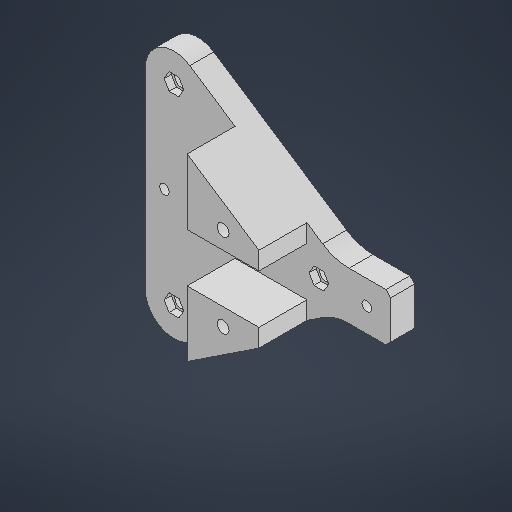
# Autodesk Inventor part: y axis something back
Saved by Autodesk Inventor 2025.1 (Build 291241000, 241)
## iProperties
Created: 2025-02-02
Part Number: y axis something back
Material: Generic
Document SubType Name: Modeling
Designer: jerem
Density: 1 g/cm^3
Appearance: Default
Author: jerem
## iProperties of the stored document y axis something back_3DPrint.ipt
Created: 2025-02-19
Part Number: y axis something back_3DPrint
Material: Generic
Document SubType Name: Modeling
Designer: jerem
Density: 1 g/cm^3
Appearance: Default
Author: jerem
Autodesk Inventor part; units mm, degrees
ref_plane "YZ Plane" through (0, 0, 0) normal (1, 0, 0) x (0, 1, 0)
ref_plane "XZ Plane" through (0, 0, 0) normal (0, 1, 0) x (-1, 0, 0)
ref_plane "XY Plane" through (0, 0, 0) normal (0, 0, 1) x (1, 0, 0)
sketch "Sketch1" plane through (0, 0, 0) normal (0, 0, 1) x (1, 0, 0)
  line L0 (0, 0) -> (30.25, 0) construction
  line L1 (0, 0) -> (-30.25, 0) construction
  line L2 (-30.25, 0) -> (-30.25, 40) construction
  line L3 (-30.25, 0) -> (-30.25, -40) construction
  circle A0 centre (-30.25, 40) radius 2.7
  circle A1 centre (-30.25, -40) radius 2.7
  circle A2 centre (30.25, 0) radius 2.7
  circle A3 centre (-30.25, 40) radius 12
  circle A4 centre (-30.25, -40) radius 12
  circle A5 centre (30.25, 0) radius 12
  line L4 (36.868172, -10.009985) -> (-23.631828, -50.009985)
  line L5 (-42.25, 40) -> (-42.25, -40)
  circle A6 centre (-34.25, 0) radius 2
  line L6 (-30.25, 0) -> (-34.25, 0) construction
  line L7 (-23.631828, 50.009985) -> (36.868172, 10.009985)
  line L8 (30.25, 0) -> (50.25, 0) construction
  circle A7 centre (50.25, 0) radius 10
  circle A8 centre (50.25, 0) radius 2
  line L9 (50.25746, 9.999997) -> (36.868172, 10.009985)
  line L10 (50.25746, -9.999997) -> (36.868172, -10.009985)
  circle A9 centre (10.25, 0) radius 2
  line L11 (50.25746, -9.999997) -> (60.257457, -9.992538)
  line L12 (60.257457, -9.992538) -> (60.242549, 9.992549)
  line L13 (60.242549, 9.992549) -> (50.25746, 9.999997)
  point P0 (-42.25, 0)
  point P1 (41.35, -4.559605)
  point P2 (41.35, 4.559605)
  point P3 (60.249997, 0.00746)
  dimension "d0" = 60.5
  dimension "d1" = 5.4
  dimension "d2" = 80
  dimension "d3" = 24
  dimension "d55" = 4
  dimension "d56" = 8
  dimension "d57" = 20
  dimension "d58" = 20
  dimension "d69" = 20
  constraints: 28 end point, 10 centre point, 10 tangent, 8 coincident, 8 point on circle, 6 equal radius, 4 horizontal, 2 collinear, 2 perpendicular, 2 vertical, 1 midpoint, 1 point on line
  measures "d0" distance of L0.end L1.end
  measures "d1" diameter of A0
  measures "d2" distance of L3.end L2.end
  measures "d3" diameter of A3
  measures "d55" diameter of A6
  measures "d56" distance of point (-42.25, 0) L6.end
  measures "d57" distance of L8.start L8.end
  measures "d58" diameter of A7
  measures "d69" distance of A9.centre L0.end
sketch "Sketch1 outline for Extrusion1" plane through (0, 0, 0) normal (0, 0, 1) x (1, 0, 0)
  arc A0 (-23.631828, 50.009985) -> (-42.25, 40) centre (-30.25, 40) ccw
  line L0 (-42.25, 40) -> (-42.25, -40)
  arc A1 (-42.25, -40) -> (-23.631828, -50.009985) centre (-30.25, -40) ccw
  line L1 (-23.631828, -50.009985) -> (36.868172, -10.009985)
  line L2 (36.868172, -10.009985) -> (60.257457, -9.992538)
  line L3 (60.257457, -9.992538) -> (60.242549, 9.992549)
  line L4 (60.242549, 9.992549) -> (36.868172, 10.009985)
  line L5 (36.868172, 10.009985) -> (-23.631828, 50.009985)
  circle A2 centre (-30.25, 40) radius 2.7
  circle A3 centre (10.25, 0) radius 2
  circle A4 centre (-34.25, 0) radius 2
  circle A5 centre (30.25, 0) radius 2.7
  circle A6 centre (-30.25, -40) radius 2.7
  circle A7 centre (50.25, 0) radius 2
extrude "Extrusion1" add sketch "Sketch1 outline for Extrusion1" against normal blind 10
fillet "Fillet1" radius 20 2 edges at (36.8682, 10.01, -5) (36.8682, -10.01, -5)
chamfer "Chamfer6" distance 2 angle 45 2 edges at (60.2425, 9.9925, -5) (60.2575, -9.9925, -5)
sketch "Sketch8" plane through (0, 0, 0) normal (0, 0, 1) x (1, 0, 0)
  line L0 (58.257457, -9.99403) -> (60.255965, -7.992538)
  line L1 (58.257457, -9.99403) -> (42.873828, -10.005505)
  arc A0 (42.873828, -10.005505) -> (31.85846, -13.322191) centre (42.888747, -30.0055) ccw
  line L2 (31.85846, -13.322191) -> (-23.631828, -50.009985)
  arc A1 (-42.25, -40) -> (-23.631828, -50.009985) centre (-30.25, -40) ccw
  line L3 (-42.25, -40) -> (-42.25, 40)
  arc A2 (-23.631828, 50.009985) -> (-42.25, 40) centre (-30.25, 40) ccw
  line L4 (-23.631828, 50.009985) -> (31.85846, 13.322191)
  arc A3 (31.85846, 13.322191) -> (42.873828, 10.005505) centre (42.888747, 30.0055) ccw
  line L5 (42.873828, 10.005505) -> (58.242549, 9.994041)
  line L6 (60.244041, 7.992549) -> (58.242549, 9.994041)
  line L7 (60.244041, 7.992549) -> (60.255965, -7.992538)
  circle A4 centre (30.25, 0) radius 2.7
  circle A5 centre (50.25, 0) radius 2
  circle A6 centre (-30.25, -40) radius 2.7
  circle A7 centre (-34.25, 0) radius 2
  circle A8 centre (10.25, 0) radius 2
  circle A9 centre (-30.25, 40) radius 2.7
  line L8 (-28.200407, -43.55) -> (-32.299593, -43.55)
  line L9 (-32.299593, -43.55) -> (-34.349187, -40)
  line L10 (-34.349187, -40) -> (-32.299593, -36.45)
  line L11 (-32.299593, -36.45) -> (-28.200407, -36.45)
  line L12 (-28.200407, -36.45) -> (-26.150813, -40)
  line L13 (-26.150813, -40) -> (-28.200407, -43.55)
  line L14 (-28.200407, 36.45) -> (-32.299593, 36.45)
  line L15 (-32.299593, 36.45) -> (-34.349187, 40)
  line L16 (-34.349187, 40) -> (-32.299593, 43.55)
  line L17 (-32.299593, 43.55) -> (-28.200407, 43.55)
  line L18 (-28.200407, 43.55) -> (-26.150813, 40)
  line L19 (-26.150813, 40) -> (-28.200407, 36.45)
  line L20 (32.299593, -3.55) -> (28.200407, -3.55)
  line L21 (28.200407, -3.55) -> (26.150813, 0)
  line L22 (26.150813, 0) -> (28.200407, 3.55)
  line L23 (28.200407, 3.55) -> (32.299593, 3.55)
  line L24 (32.299593, 3.55) -> (34.349187, 0)
  line L25 (34.349187, 0) -> (32.299593, -3.55)
  point P0 (0, 0)
  dimension "d83" = 7.1
  dimension "d84" = 7.1
  dimension "d85" = 7.1
  constraints: 36 end point, 3 coincident, 3 horizontal, 39 other
  measures "d83" distance between parallel lines of L23 L20
  measures "d84" distance between parallel lines of L17 L14
  measures "d85" distance between parallel lines of L11 L8
extrude "Extrusion9" cut sketch "Sketch8" against normal blind 3 contours L8 L9 L10 L11 L12 L13 | L14 L15 L16 L17 L18 L19 | L20 L21 L22 L23 L24 L25
sketch "Sketch5" plane through (0, 0, 0) normal (0, 0, 1) x (1, 0, 0)
  arc A0 (-42.25, -40) -> (-23.631828, -50.009985) centre (-30.25, -40) ccw
  line L0 (-23.631828, -50.009985) -> (31.85846, -13.322191)
  arc A1 (42.873828, -10.005505) -> (31.85846, -13.322191) centre (42.888747, -30.0055) ccw
  line L1 (42.873828, -10.005505) -> (58.257457, -9.99403)
  arc A2 (31.85846, 13.322191) -> (42.873828, 10.005505) centre (42.888747, 30.0055) ccw
  line L2 (31.85846, 13.322191) -> (-23.631828, 50.009985)
  arc A3 (-23.631828, 50.009985) -> (-42.25, 40) centre (-30.25, 40) ccw
  line L3 (-42.25, 40) -> (-42.25, -40)
  circle A4 centre (-34.25, 0) radius 2
  circle A5 centre (50.25, 0) radius 2
  line L4 (-4.75, 10.2) -> (-4.75, 37.526132)
  line L5 (-4.75, 10.2) -> (25.25, 10.2)
  line L6 (25.25, 10.2) -> (25.25, 17.691421)
  line L7 (60.255965, -7.992538) -> (60.244041, 7.992549)
  line L8 (58.242549, 9.994041) -> (42.873828, 10.005505)
  line L9 (60.255965, -7.992538) -> (58.257457, -9.99403)
  line L10 (58.242549, 9.994041) -> (60.244041, 7.992549)
  dimension "d66" = 30
  dimension "d92" = 10.2
  dimension "d93" = 25
  constraints: 6 end point, 2 point on line, 1 horizontal, 1 perpendicular, 1 vertical, 1 other
  measures "d66" distance of L4.start L5.end
  measures "d92" distance from line of L5 A5.centre
  measures "d93" distance from line of A5.centre L6
extrude "Extrusion6" add sketch "Sketch5" along normal blind 20 contours L2 L6 L5 L4
sketch "Sketch9" plane through (0, 0, 20) normal (0, 0, 1) x (1, 0, 0)
  circle A0 centre (10.25, 0) radius 2
  line L0 (25.25, 10.2) -> (25.25, 17.691421)
  line L1 (25.25, 17.691421) -> (-4.75, 37.526132)
  line L2 (-4.75, 37.526132) -> (-4.75, 10.2)
  line L3 (-4.75, 10.2) -> (25.25, 10.2)
  line L4 (10.25, 0) -> (10.25, 17.5) construction
  circle A1 centre (10.25, 17.5) radius 2.5
  point P0 (0, 0)
  dimension "d88" = 17.5
  dimension "d89" = 5
  constraints: 2 end point, 1 centre point, 1 coincident, 1 vertical
  measures "d88" distance of L4.start L4.end
  measures "d89" diameter of A1
extrude "Extrusion10" cut sketch "Sketch9" against normal blind 5 contours A1
mirror "Mirror1" about plane through (0, 0, 0) normal (0, 1, 0) of "Extrusion10", "Extrusion6"
equation "\"d84\" = d83"
equation "\"d85\" = d83"
equation "\"b\" = 2"
body "Solid1"
